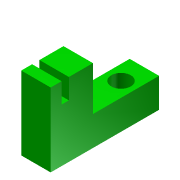
# Autodesk Inventor part: grip1
Saved by Autodesk Inventor 2011 (Build 150239000, 239)
## iProperties
Created: 2011-06-13
Part Number: grip1
Document SubType Name: Modeling
Designer: ijs09
Density: 1 g/cm^3
Author: ijs09
Autodesk Inventor part; units mm, degrees
ref_plane "YZ Plane" through (0, 0, 0) normal (1, 0, 0) x (0, 1, 0)
ref_plane "XZ Plane" through (0, 0, 0) normal (0, 1, 0) x (-1, 0, 0)
ref_plane "XY Plane" through (0, 0, 0) normal (0, 0, 1) x (1, 0, 0)
sketch "Sketch2" plane through (0, 0, 0) normal (1, 0, 0) x (0, 1, 0)
  line L0 (-8.2712, 10.508) -> (-8.2712, 5.008)
  line L1 (-8.2712, 5.008) -> (-10.2712, 5.008)
  line L2 (-10.2712, 5.008) -> (-10.2712, 10.508)
  line L3 (-10.2712, 10.508) -> (-13.2312, 10.508)
  line L4 (-13.2312, 10.508) -> (-13.2312, -9.492)
  line L5 (-13.2312, -9.492) -> (16.2688, -9.492)
  line L6 (16.2688, -1.492) -> (-1.7312, -1.492)
  line L7 (-1.7312, -1.492) -> (-1.7312, 10.508)
  line L8 (16.2688, -9.492) -> (16.2688, -1.492)
  line L9 (-1.7312, 10.508) -> (-8.2712, 10.508)
  point P0 (0, 0)
  dimension "d2" = 2
  dimension "d3" = 5.5
  dimension "d4" = 20
  dimension "d9" = 12
  dimension "d10" = 29.5
  dimension "d11" = 24.54
  dimension "d12" = 18
  constraints: 20 end point, 2 parallel, 1 perpendicular
  measures "d2" distance between parallel lines of L2 L0
  measures "d3" distance between parallel lines of L1 L3
  measures "d4" distance between parallel lines of L5 L3
  measures "d9" distance between parallel lines of L9 L6
  measures "d10" distance between parallel lines of L8 L4
  measures "d11" distance between parallel lines of L0 L8
  measures "d12" distance between parallel lines of L8 L7
extrude "Extrusion1" add sketch "Sketch2" along normal blind 8
sketch "Sketch3" plane through (0, -1.7312, -1.492) normal (0, 0, 1) x (1, 0, 0)
  line L0 (0, 18) -> (8, 18) projected
  line L1 (0, 0) -> (0, 18) projected
  point P0 (0, 1.7312)
  point P1 (4, 11.65)
  dimension "d13" = 6.35
  dimension "d14" = 4
  measures "d13" distance from line of L0 point (4, 11.65)
  measures "d14" distance from line of L1 point (4, 11.65)
hole "Hole1" at (4, 9.9188, -1.492) direction (0, 0, -1) diameter 5.3 depth 8 tip angle 118
equation "\"d4\" = d1"
equation "\"d1\" = 20"
body "Solid1"
